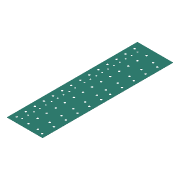
# Autodesk Inventor part: 17-0028-0027
Saved by Autodesk Inventor 2016 SP2 (Build 200236200, 236)
## iProperties
Category: IOP
Company: Universiteit van Amsterdam
Created: 2017-11-10
Part Number: 17-0028-0027
Material: Generic
Document SubType Name: Modeling
Designer: Daan Giesen
Density: 1 g/cm^3
Appearance: RAL 5018 Turqoise blue
Mass: 4.38818 g
Surface Area: 441.964 cm^2
Volume: 4.38818 cm^3
Project: Digital PID Loop
Cost Center: 17-0028
User Status: Work in Progress
Authority: Reichsöllner, Lukas
Description: Insulating layer
Author: Daan Giesen
Title: Digital PID Loop
Revision Number: A
Autodesk Inventor part; units mm, degrees
ref_plane "YZ Plane" through (0, 0, 0) normal (1, 0, 0) x (0, 1, 0)
ref_plane "XZ Plane" through (0, 0, 0) normal (0, 1, 0) x (-1, 0, 0)
ref_plane "XY Plane" through (0, 0, 0) normal (0, 0, 1) x (1, 0, 0)
sketch "Sketch1" plane through (0, 0, 0) normal (0, 0, 1) x (1, 0, 0)
  line L0 (0, 201.6) -> (0, -201.6) construction
  circle A0 centre (17.361, 111.95) radius 2 construction
  circle A1 centre (17.361, 85.95) radius 2 construction
  circle A2 centre (17.361, 59.95) radius 2 construction
  circle A3 centre (17.361, 33.95) radius 2 construction
  circle A4 centre (17.361, 7.95) radius 2 construction
  circle A5 centre (17.361, -25.35) radius 2 construction
  circle A6 centre (17.361, -51.35) radius 2 construction
  circle A7 centre (17.361, -77.35) radius 2 construction
  circle A8 centre (17.361, -103.35) radius 2 construction
  circle A9 centre (17.361, -129.35) radius 2 construction
  circle A10 centre (17.361, -116.35) radius 2 construction
  circle A11 centre (17.361, -90.35) radius 2 construction
  circle A12 centre (17.361, -64.35) radius 2 construction
  circle A13 centre (17.361, -38.35) radius 2 construction
  circle A14 centre (17.361, -12.35) radius 2 construction
  circle A15 centre (17.361, 20.95) radius 2 construction
  circle A16 centre (17.361, 46.95) radius 2 construction
  circle A17 centre (17.361, 72.95) radius 2 construction
  circle A18 centre (17.361, 98.95) radius 2 construction
  circle A19 centre (17.361, 124.95) radius 2 construction
  circle A20 centre (8, -12) radius 2.65 construction
  circle A21 centre (8, -52) radius 2.65 construction
  circle A22 centre (8, -92) radius 2.65 construction
  circle A23 centre (8, -132) radius 2.65 construction
  circle A24 centre (34, -112) radius 2.65 construction
  circle A25 centre (34, -72) radius 2.65 construction
  circle A26 centre (34, -32) radius 2.65 construction
  circle A27 centre (34, 8) radius 2.65 construction
  circle A28 centre (34, 48) radius 2.65 construction
  circle A29 centre (8, 28) radius 2.65 construction
  circle A30 centre (8, 68) radius 2.65 construction
  circle A31 centre (8, 88) radius 2.65 construction
  circle A32 centre (8, 108) radius 2.65 construction
  circle A33 centre (8, 128) radius 2.65 construction
  circle A34 centre (68, 118) radius 2.65 construction
  circle A35 centre (55, 95.7) radius 2.65 construction
  circle A36 centre (55, 69.7) radius 2.65 construction
  circle A37 centre (55, 43.7) radius 2.65 construction
  circle A38 centre (55, 17.7) radius 2.65 construction
  circle A39 centre (55, -2.3) radius 2.65 construction
  circle A40 centre (55, -28.3) radius 2.65 construction
  circle A41 centre (55, -54.3) radius 2.65 construction
  circle A42 centre (55, -80.3) radius 2.65 construction
  circle A43 centre (55, -106.3) radius 2.65 construction
  circle A44 centre (55, -132.3) radius 2.65 construction
  circle A45 centre (68, -136) radius 2.65 construction
  circle A46 centre (68, -110) radius 2.65 construction
  circle A47 centre (68, -84) radius 2.65 construction
  circle A48 centre (68, -58) radius 2.65 construction
  circle A49 centre (68, -32) radius 2.65 construction
  circle A50 centre (68, -6) radius 2.65 construction
  circle A51 centre (68, 14) radius 2.65 construction
  circle A52 centre (68, 40) radius 2.65 construction
  circle A53 centre (68, 66) radius 2.65 construction
  circle A54 centre (68, 92) radius 2.65 construction
  circle A55 centre (55, 121.7) radius 2.65 construction
  circle A56 centre (34, 128) radius 2.65 construction
  circle A57 centre (34, 108) radius 2.65 construction
  circle A58 centre (34, 88) radius 2.65 construction
  circle A59 centre (8, 48) radius 2.65 construction
  circle A60 centre (34, 68) radius 2.65 construction
  circle A61 centre (34, 28) radius 2.65 construction
  circle A62 centre (34, -12) radius 2.65 construction
  circle A63 centre (34, -52) radius 2.65 construction
  circle A64 centre (34, -92) radius 2.65 construction
  circle A65 centre (34, -132) radius 2.65 construction
  circle A66 centre (8, -112) radius 2.65 construction
  circle A67 centre (8, -72) radius 2.65 construction
  circle A68 centre (8, -32) radius 2.65 construction
  circle A69 centre (8, 8) radius 2.65 construction
  line L1 (75, 142) -> (75, -142) projected
  line L2 (0, 142) -> (75, 142) projected
  line L3 (0, -142) -> (0, 142) projected
  line L4 (75, -142) -> (0, -142) construction
  line L5 (-2, -144) -> (-2, 144)
  line L6 (-2, 144) -> (77, 144)
  line L7 (77, 144) -> (77, -144)
  line L8 (77, -144) -> (-2, -144)
  circle A70 centre (8, -132) radius 2.05
  circle A71 centre (8, -112) radius 2.05
  circle A72 centre (8, -92) radius 2.05
  circle A73 centre (8, -72) radius 2.05
  circle A74 centre (8, -52) radius 2.05
  circle A75 centre (8, -32) radius 2.05
  circle A76 centre (8, -12) radius 2.05
  circle A77 centre (8, 8) radius 2.05
  circle A78 centre (8, 28) radius 2.05
  circle A79 centre (8, 48) radius 2.05
  circle A80 centre (8, 68) radius 2.05
  circle A81 centre (8, 88) radius 2.05
  circle A82 centre (8, 108) radius 2.05
  circle A83 centre (8, 128) radius 2.05
  circle A84 centre (17.361, 124.95) radius 1.55
  circle A85 centre (17.361, 111.95) radius 1.55
  circle A86 centre (17.361, 98.95) radius 1.55
  circle A87 centre (17.361, 85.95) radius 1.55
  circle A88 centre (17.361, 72.95) radius 1.55
  circle A89 centre (17.361, 59.95) radius 1.55
  circle A90 centre (17.361, 46.95) radius 1.55
  circle A91 centre (17.361, 33.95) radius 1.55
  circle A92 centre (17.361, 20.95) radius 1.55
  circle A93 centre (17.361, 7.95) radius 1.55
  circle A94 centre (17.361, -12.35) radius 1.55
  circle A95 centre (17.361, -25.35) radius 1.55
  circle A96 centre (17.361, -38.35) radius 1.55
  circle A97 centre (17.361, -51.35) radius 1.55
  circle A98 centre (17.361, -64.35) radius 1.55
  circle A99 centre (17.361, -77.35) radius 1.55
  circle A100 centre (17.361, -90.35) radius 1.55
  circle A101 centre (17.361, -103.35) radius 1.55
  circle A102 centre (17.361, -116.35) radius 1.55
  circle A103 centre (17.361, -129.35) radius 1.55
  circle A104 centre (34, -132) radius 2.05
  circle A105 centre (34, -112) radius 2.05
  circle A106 centre (34, -92) radius 2.05
  circle A107 centre (34, -72) radius 2.05
  circle A108 centre (34, -52) radius 2.05
  circle A109 centre (34, -32) radius 2.05
  circle A110 centre (34, -12) radius 2.05
  circle A111 centre (34, 8) radius 2.05
  circle A112 centre (34, 28) radius 2.05
  circle A113 centre (34, 48) radius 2.05
  circle A114 centre (34, 68) radius 2.05
  circle A115 centre (34, 88) radius 2.05
  circle A116 centre (34, 108) radius 2.05
  circle A117 centre (34, 128) radius 2.05
  circle A118 centre (55, 121.7) radius 2.05
  circle A119 centre (68, 118) radius 2.05
  circle A120 centre (55, 95.7) radius 2.05
  circle A121 centre (68, 92) radius 2.05
  circle A122 centre (55, 69.7) radius 2.05
  circle A123 centre (68, 66) radius 2.05
  circle A124 centre (55, 43.7) radius 2.05
  circle A125 centre (55, 17.7) radius 2.05
  circle A126 centre (68, 40) radius 2.05
  circle A127 centre (68, 14) radius 2.05
  circle A128 centre (55, -2.3) radius 2.05
  circle A129 centre (68, -6) radius 2.05
  circle A130 centre (55, -28.3) radius 2.05
  circle A131 centre (68, -32) radius 2.05
  circle A132 centre (55, -54.3) radius 2.05
  circle A133 centre (68, -58) radius 2.05
  circle A134 centre (55, -80.3) radius 2.05
  circle A135 centre (55, -106.3) radius 2.05
  circle A136 centre (68, -84) radius 2.05
  circle A137 centre (68, -110) radius 2.05
  circle A138 centre (55, -132.3) radius 2.05
  circle A139 centre (68, -136) radius 2.05
  dimension "d10" = 2
  dimension "d11" = 4.1
  dimension "d12" = 3.1
  constraints: 70 centre point, 68 equal radius, 8 end point, 3 other
  measures "d10" distance between parallel lines of L8 L4
  measures "d11" diameter of A70
  measures "d12" diameter of A103
extrude "Extrusion4" add sketch "Sketch1" along normal blind 0.2
body "Solid4"
